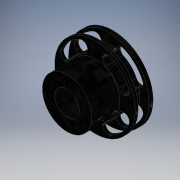
# Autodesk Inventor part: core
Saved by Autodesk Inventor 2019.4 (Build 234330000, 330)
## iProperties
Created: 2019-10-01
Part Number: core
Material: Generic
Document SubType Name: Modeling
Designer: cdi
Density: 1 g/cm^3
Appearance: Black
Author: cdi
Autodesk Inventor part; units mm, degrees
ref_plane "YZ Plane" through (0, 0, 0) normal (1, 0, 0) x (0, 1, 0)
ref_plane "XZ Plane" through (0, 0, 0) normal (0, 1, 0) x (-1, 0, 0)
ref_plane "XY Plane" through (0, 0, 0) normal (0, 0, 1) x (1, 0, 0)
sketch "Sketch1" plane through (0, 0, 0) normal (0, 0, 1) x (1, 0, 0)
  circle A0 centre (0, 0) radius 12
  circle A1 centre (0, 0) radius 6
  dimension "d0" = 24
  dimension "d1" = 12
  constraints: 2 centre point, 2 coincident
  measures "d0" diameter of A0
  measures "d1" diameter of A1
extrude "Extrusion1" add sketch "Sketch1" along normal blind 10
sketch "Sketch2" plane through (0, 0, 0) normal (0, 0, -1) x (-1, 0, 0)
  circle A0 centre (0, 0) radius 6 projected
  circle A1 centre (0, 0) radius 12 projected
extrude "Extrusion2" add sketch "Sketch2" along normal blind 4
sketch "Sketch3" plane through (0, 0, -4) normal (0, 0, -1) x (-1, 0, 0)
  circle A0 centre (0, 0) radius 19.5
  circle A1 centre (0, 0) radius 6 projected
  dimension "d20" = 360
  dimension "d6" = 39
  constraints: 1 centre point, 1 coincident
  measures "d6" diameter of A0
extrude "Extrusion3" add sketch "Sketch3" along normal blind 1.5
sketch "Sketch4" plane through (0, 0, -5.5) normal (0, 0, -1) x (-1, 0, 0)
  circle A0 centre (0, 0) radius 15
  circle A1 centre (0, 0) radius 6 projected
  circle A2 centre (0, 0) radius 19.5 projected
  dimension "d9" = 30
  constraints: 1 centre point, 1 coincident
  measures "d9" diameter of A0
extrude "Extrusion4" add sketch "Sketch4" along normal blind 5.2 contours A0
sketch "Sketch5" plane through (0, 0, -10.7) normal (0, 0, -1) x (-1, 0, 0)
  circle A0 centre (0, 0) radius 6 projected
  circle A1 centre (0, 0) radius 19.5 projected
extrude "Extrusion5" add sketch "Sketch5" along normal blind 2
sketch "Sketch6" plane through (0, 0, -12.7) normal (0, 0, -1) x (-1, 0, 0)
  line L0 (0, 0) -> (0, 10.6)
  line L1 (0.9, 0) -> (0.9, 10.6)
  line L2 (-0.9, 0) -> (-0.9, 10.6)
  line L3 (0, 0.9) -> (-10.6, 0.9)
  line L4 (0, -0.9) -> (-10.6, -0.9)
  line L5 (-0.9, 0) -> (-0.9, -10.6)
  line L6 (0.9, 0) -> (0.9, -10.6)
  line L7 (0, -0.9) -> (10.6, -0.9)
  line L8 (0, 0.9) -> (10.6, 0.9)
  arc A0 (0, 10.6) -> (10.5617, -0.9) centre (0, 0) ccw
  arc A1 (10.5617, 0.9) -> (0.9, 10.5617) centre (0, 0) ccw
  arc A2 (7.0427, 0.9) -> (0.9, 7.0427) centre (0, 0) ccw
  arc A3 (0, 7.1) -> (7.0427, -0.9) centre (0, 0) ccw
  dimension "d16" = 1.8
  dimension "d17" = 0.9
  dimension "d20" = 360
  constraints: 18 end point, 8 point on circle, 7 point on line, 4 centre point, 2 coincident, 2 parallel, 1 vertical, 25 other
  measures "d16" distance between parallel lines of L2 L1
  measures "d17" distance between parallel lines of L0 L1
extrude "Extrusion6" cut sketch "Sketch6" against normal blind 7 contours L1 A1 L8 A2
fillet "Fillet1" radius 1.7 4 edges at (-0.9, 10.5617, -9.2) (-0.9, 7.0427, -9.2) (-10.5617, 0.9, -9.2) (-7.0427, 0.9, -9.2)
pattern_circular "Circular Pattern1" count 4 over 360 about axis through (0, 0, 0) along (0, 0, 1) of "Extrusion6", "Fillet1"
sketch "Sketch7" plane through (0, 0, -12.7) normal (0, 0, -1) x (-1, 0, 0)
  circle A0 centre (0, 0) radius 12.5
  circle A1 centre (0, 12.5) radius 1.5
  dimension "d28" = 25
  dimension "d29" = 3
  constraints: 1 centre point, 1 coincident, 1 vertical alignment, 2 other
  measures "d29" diameter of A1
hole "Hole1" at (0, 12.5, -12.7) direction (0, 0, 1) diameter 2.459 depth 8 thread size "M3x0.5" class "6H" standard "ISO Metric profile"
pattern_circular "Circular Pattern2" count 4 over 360 about axis through (0, 0, 0) along (0, 0, 1) of "Hole1"
sketch "Sketch8" plane through (0, 0, -12.7) normal (0, 0, -1) x (-1, 0, 0)
  arc A0 (6.783, 2.0977) -> (8.4071, 0.9) centre (8.4071, 2.6) ccw projected
  line L0 (8.5118, 0.9) -> (8.4071, 0.9) projected
  arc A1 (8.5118, 0.9) -> (10.1376, 3.0966) centre (8.5118, 2.6) ccw projected
  arc A2 (10.1376, 3.0966) -> (3.0966, 10.1376) centre (0, 0) ccw projected
  arc A3 (3.0966, 10.1376) -> (0.9, 8.5118) centre (2.6, 8.5118) ccw projected
  line L1 (0.9, 8.4071) -> (0.9, 8.5118) projected
  arc A4 (0.9, 8.4071) -> (2.0977, 6.783) centre (2.6, 8.4071) ccw projected
  arc A5 (6.783, 2.0977) -> (2.0977, 6.783) centre (0, 0) ccw projected
  line L2 (0, 0) -> (20.618, 0)
  line L3 (0, 3.65) -> (20.618, 3.65)
  line L4 (0, -3.65) -> (20.618, -3.65)
  line L5 (-3.65, 0) -> (-3.65, 20.618)
  line L6 (3.65, 0) -> (3.65, 20.618)
  line L7 (0, -3.65) -> (-20.618, -3.65)
  line L8 (0, 3.65) -> (-20.618, 3.65)
  line L9 (3.65, 0) -> (3.65, -20.618)
  line L10 (-3.65, 0) -> (-3.65, -20.618)
  arc A6 (17.626, 3.65) -> (-3.65, -17.626) centre (0, 0) ccw
  arc A7 (3.65, -17.626) -> (17.626, -3.65) centre (0, 0) ccw
  arc A8 (3.65, -11.9552) -> (11.9552, -3.65) centre (0, 0) ccw
  arc A9 (12.5, 0) -> (-3.65, -11.9552) centre (0, 0) ccw
  dimension "d42" = 7.3
  dimension "d43" = 3.65
  dimension "d46" = 360
  constraints: 18 end point, 8 point on circle, 8 point on line, 4 centre point, 2 coincident, 2 parallel, 1 horizontal, 25 other
  measures "d42" distance between parallel lines of L3 L4
  measures "d43" distance between parallel lines of L2 L4
extrude "Extrusion7" cut sketch "Sketch8" against normal up to surface (8.7 mm away) contours L4 A7 L9 A8
fillet "Fillet2" radius 2.6 6 edges at (-17.626, -3.65, -11.7) (-17.626, -3.65, -4.75) (-11.9552, -3.65, -8.35) (-3.65, -11.9552, -8.35) (-3.65, -17.626, -11.7) (-3.65, -17.626, -4.75)
pattern_circular "Circular Pattern3" count 4 over 360 about axis through (0, 0, 0) along (0, 0, 1) of "Extrusion7", "Fillet2"
equation "\"d17\" = 0.5 * d16"
equation "\"d43\" = 0.5 * d42"
body "Solid1"
